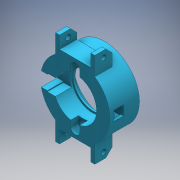
# Autodesk Inventor part: Tracking Bracelet
Saved by Autodesk Inventor 2016 (Build 200138000, 138)
## iProperties
Created: 2016-04-05
Part Number: Tracking Bracelet
Material: ABS Plastic
Document SubType Name: Modeling
Designer: xdlea
Density: 1.06 g/cm^3
Appearance: Turquoise
Author: xdlea
Autodesk Inventor part; units mm, degrees
ref_plane "YZ Plane" through (0, 0, 0) normal (1, 0, 0) x (0, 1, 0)
sketch "Sketch1" plane through (0, 0, 0) normal (0, 1, 0) x (-1, 0, 0)
  arc A0 (21.65, 4.5) -> (21.65, -4.5) centre (0, 0) ccw
  arc A1 (11.401069, 5.125) -> (11.401069, -5.125) centre (0, 0) ccw
  arc A2 (12.624381, 5.125) -> (12.624381, -5.125) centre (0, 0) ccw
  circle A3 centre (0, 0) radius 11.25 construction
  line L0 (10.014833, 5.125) -> (17.75, 5.125) construction
  line L1 (17.75, 5.125) -> (17.75, -5.125) construction
  line L2 (17.75, -5.125) -> (10.014833, -5.125) construction
  line L3 (10.014833, -5.125) -> (10.014833, 5.125) construction
  line L4 (17.75, 4.5) -> (21.65, 4.5) construction
  line L5 (21.65, 4.5) -> (21.65, -4.5) construction
  line L6 (21.65, -4.5) -> (17.75, -4.5) construction
  line L7 (17.75, -4.5) -> (17.75, 4.5) construction
  line L8 (-30.957812, 0) -> (30.957812, 0) construction
  arc A4 (19.602847, 4.5) -> (19.602847, -4.5) centre (0, 0) ccw
  line L9 (12.624381, 5.125) -> (17.75, 5.125)
  line L10 (17.75, 5.125) -> (17.75, 4.5)
  line L11 (17.75, 4.5) -> (19.602847, 4.5)
  line L12 (19.602847, 4.5) -> (21.65, 4.5)
  line L13 (21.65, -4.5) -> (19.602847, -4.5)
  line L14 (19.602847, -4.5) -> (17.75, -4.5)
  line L15 (17.75, -4.5) -> (17.75, -5.125)
  line L16 (17.75, -5.125) -> (12.624381, -5.125)
  line L17 (12.624381, 5.125) -> (11.401069, 5.125)
  line L18 (12.624381, -5.125) -> (11.401069, -5.125)
  arc A5 (11.401069, -5.125) -> (11.401069, 5.125) centre (0, 0) ccw
  arc A6 (12.624381, -5.125) -> (12.624381, 5.125) centre (0, 0) ccw
  arc A7 (19.602847, -4.5) -> (19.602847, 4.5) centre (0, 0) ccw
  arc A8 (21.65, -4.5) -> (21.65, 4.5) centre (0, 0) ccw
  line L19 (-21.908275, -3) -> (-19.908275, -3)
  line L20 (-19.908275, -3) -> (-19.908275, 3)
  line L21 (-19.908275, 3) -> (-21.908275, 3)
  line L22 (-21.908275, 3) -> (-21.908275, -3)
  line L23 (-19.908275, -4.6077) -> (-14.836045, -4.6077)
  line L24 (-14.836045, -4.6077) -> (-14.836045, 2.3923)
  line L25 (-14.836045, 2.3923) -> (-19.908275, 2.3923)
  line L26 (-19.908275, 2.3923) -> (-19.908275, -4.6077)
  dimension "d1" = 25
  dimension "d4" = 27.25
  dimension "d7" = 22.5
  dimension "d8" = 29
  dimension "d9" = 10.25
  dimension "d10" = 3.9
  dimension "d11" = 9
  dimension "d12" = 2
  dimension "d51" = 6
  dimension "d52" = 2
  dimension "d53" = 7
  constraints: 52 end point, 20 point on circle, 9 centre point, 8 parallel, 7 point on line, 6 coincident, 6 perpendicular, 4 horizontal, 3 collinear, 3 concentric, 1 other
  measures "d1" diameter of A1
  measures "d4" diameter of A2
  measures "d7" diameter of A3
  measures "d9" distance of L0.end L1.end
  measures "d10" distance of L5.end L6.end
  measures "d11" distance of L5.end L4.end
  measures "d12" radial gap between concentric circles of A0 A4
  measures "d51" distance between parallel lines of L21 L19
  measures "d52" distance of L19.start L19.end
  measures "d53" distance between parallel lines of L25 L23
sketch "Sketch1 outline for Extrusion3" plane through (0, 0, 0) normal (0, 1, 0) x (-1, 0, 0)
  circle A0 centre (0, 0) radius 22.112723
  circle A1 centre (0, 0) radius 20.112723
extrude "Extrusion3" add sketch "Sketch1 outline for Extrusion3" along normal blind 7.6
sketch "Sketch1 outline for Extrusion4" plane through (0, 0, 0) normal (0, 1, 0) x (-1, 0, 0)
  circle A0 centre (0, 0) radius 12.5
  circle A1 centre (0, 0) radius 20.112723
extrude "Extrusion4" add sketch "Sketch1 outline for Extrusion4" along normal blind 1.25
sketch "Sketch1 outline for Extrusion5" plane through (0, 0, 0) normal (0, 1, 0) x (-1, 0, 0)
  arc A0 (21.65, 4.5) -> (21.65, -4.5) centre (0, 0) ccw
  line L0 (21.65, -4.5) -> (17.75, -4.5)
  line L1 (17.75, -4.5) -> (17.75, -5.125)
  line L2 (17.75, -5.125) -> (12.624381, -5.125)
  arc A1 (12.624381, -5.125) -> (12.624381, 5.125) centre (0, 0) cw
  line L3 (12.624381, 5.125) -> (17.75, 5.125)
  line L4 (17.75, 5.125) -> (17.75, 4.5)
  line L5 (17.75, 4.5) -> (21.65, 4.5)
extrude "Extrusion5" add sketch "Sketch1 outline for Extrusion5" against normal blind 11.25
sketch "Sketch1 outline for Extrusion6" plane through (0, 0, 0) normal (0, 1, 0) x (-1, 0, 0)
  arc A0 (21.65, -4.5) -> (21.65, 4.5) centre (0, 0) ccw
  line L0 (21.65, 4.5) -> (17.75, 4.5)
  line L1 (17.75, 4.5) -> (17.75, 5.125)
  line L2 (17.75, 5.125) -> (12.624381, 5.125)
  arc A1 (12.624381, 5.125) -> (12.624381, -5.125) centre (0, 0) cw
  line L3 (12.624381, -5.125) -> (17.75, -5.125)
  line L4 (17.75, -5.125) -> (17.75, -4.5)
  line L5 (17.75, -4.5) -> (21.65, -4.5)
extrude "Extrusion6" add sketch "Sketch1 outline for Extrusion6" against normal blind 1
sketch "Sketch2" plane through (0, 1.25, 0) normal (0, 1, 0) x (1, 0, 0)
  circle A0 centre (0, 17) radius 2.425
  line L0 (30.957812, 0) -> (-30.957812, 0) construction
  line L1 (0, 42.7) -> (0, -42.7) construction
  point P0 (0, 0)
  dimension "d21" = 4.85
  dimension "d22" = 17
  constraints: 1 centre point, 1 point on line
  measures "d21" diameter of A0
  measures "d22" distance from line of L0 A0.centre
sketch "Sketch2 outline for Extrusion7" plane through (0, 1.25, 0) normal (0, 1, 0) x (1, 0, 0)
  circle A0 centre (0, 17) radius 2.425
extrude "Extrusion7" cut sketch "Sketch2 outline for Extrusion7" against normal blind 7.5
sketch "Sketch3" plane through (0, -6.25, -17) normal (0, 1, 0) x (1, 0, 0)
  arc A0 (2.875, 0) -> (-2.875, 0) centre (0, 0) ccw
  circle A1 centre (0, -34) radius 2.425
  circle A2 centre (0, 0) radius 2.425
  line L0 (-2.875, 0) -> (-2.875, -3.681779)
  arc A3 (-12.624381, -22.125) -> (-12.624381, -11.875) centre (0, -17) ccw
  line L1 (2.875, 0) -> (2.875, -3.681779)
  arc A4 (2.875, -3.681779) -> (-2.875, -3.681779) centre (0, -17) ccw
  dimension "d25" = 5.75
  constraints: 6 point on circle, 4 end point, 2 centre point, 2 concentric, 2 tangent, 1 parallel, 1 vertical
  measures "d25" diameter of A0
sketch "Sketch3 outline for Extrusion8" plane through (0, -6.25, -17) normal (0, 1, 0) x (1, 0, 0)
  arc A0 (2.875, 0) -> (-2.875, 0) centre (0, 0) ccw
  line L0 (2.875, -3.681779) -> (2.875, 0)
  arc A1 (-2.875, -3.681779) -> (2.875, -3.681779) centre (0, -17) cw
  line L1 (-2.875, 0) -> (-2.875, -3.681779)
extrude "Extrusion8" cut sketch "Sketch3 outline for Extrusion8" against normal blind 7.5
chamfer "Chamfer1" distance 3 angle 25 1 edges at (-2.425, 1.25, -17)
sketch "Sketch5" plane through (0, 0, 0) normal (1, 0, 0) x (0, 1, 0)
  line L0 (0, 42.7) -> (0, -42.7) construction
  line L1 (-48.962855, 0) -> (11.753777, 0) construction
  ellipse E0 centre (-14.482928, 0) end of major axis (3.017072, 0) minor radius 22.5 (-11.25, 22.112723) -> (-11.25, -22.112723) ccw
  line L2 (-11.25, 22.112723) -> (-11.25, -22.112723) construction
  ellipse E1 centre (-14.482928, 0) end of major axis (-14.482928, 30.5) minor radius 25.5 (3.079973, 22.112723) -> (3.079973, -22.112723) ccw
  line L3 (3.079973, -22.112723) -> (-11.25, -22.112723)
  line L4 (-11.25, 22.112723) -> (3.079973, 22.112723)
  spline S0 degree 5 poles (-9.370672, 29.888789) (-9.607667, 29.946061) (-9.845455, 30.000062) (-10.08398, 30.050769) (-13.432172, 30.714105) (-16.900715, 30.723992) (-20.090193, 30.119162) (-26.095525, 27.802909) (-31.037596, 23.674589) (-33.16656, 21.251032) (-36.759867, 15.847694) (-38.905719, 9.719856) (-39.623591, 6.515342) (-40.342276, 0) (-39.623591, -6.515342) (-38.905719, -9.719856) (-36.759867, -15.847694) (-33.16656, -21.251032) (-31.037596, -23.674589) (-26.095525, -27.802909) (-20.090193, -30.119162) (-16.900715, -30.723992) (-13.432172, -30.714105) (-10.08398, -30.050769) (-9.845455, -30.000062) (-9.607667, -29.946061) (-9.370672, -29.888789) knots 0 0 0 0 0 0 0.01237227 0.01237227 0.01237227 0.17318041 0.17318041 0.17318041 0.33468989 0.33468989 0.33468989 0.5 0.5 0.5 0.66531011 0.66531011 0.66531011 0.82681959 0.82681959 0.82681959 0.98762773 0.98762773 0.98762773 1 1 1 1 1 1 construction
  point P0 (0, 0)
  point P1 (-11.25, -4.5)
  point P2 (-11.25, 4.5)
  dimension "d39" = 8
  dimension "d40" = 22.5
  dimension "d41" = 17.5
  dimension "d42" = 30.5
  dimension "d43" = 25.5
  constraints: 4 end point, 3 point on line, 1 coincident, 1 parallel, 1 perpendicular, 1 vertical alignment, 13 other
pattern_circular "Circular Pattern2" count 2 over 360 about axis through (0, 0, 0) along (0, -1, 0) of "Extrusion7", "Extrusion8", "Chamfer1"
ref_plane "Work Plane1" through (22.112723, 0, 0) normal (1, 0, 0) x (0, 1, 0)
sketch "Sketch8" plane through (22.112723, 0, 0) normal (1, 0, 0) x (0, 1, 0)
  line L0 (-8.575, 3.075) -> (-2.425, 3.075)
  line L1 (-2.425, 3.075) -> (-2.425, -3.075)
  line L2 (-2.425, -3.075) -> (-8.575, -3.075)
  line L3 (-8.575, -3.075) -> (-8.575, 3.075)
  line L4 (-8.575, 3.075) -> (-2.425, -3.075) construction
  line L5 (-2.425, 3.075) -> (-8.575, -3.075) construction
  line L6 (-15.02, 0) -> (11.37, 0) construction
  line L7 (0, 30.957812) -> (0, -30.957812) construction
  point P0 (0, 0)
  point P1 (-5.5, 0)
  dimension "d54" = 6.15
  dimension "d55" = 6.15
  dimension "d56" = 5.5
  constraints: 12 end point, 2 midpoint, 2 parallel, 1 horizontal, 1 perpendicular, 1 point on line
  measures "d54" distance of L0.end L1.end
  measures "d55" distance of L1.end L2.end
  measures "d56" distance from line of point (-5.5, 0) L7
sketch "Sketch8 outline for Extrusion11" plane through (22.112723, 0, 0) normal (1, 0, 0) x (0, 1, 0)
  line L0 (-8.575, 3.075) -> (-2.425, 3.075)
  line L1 (-2.425, 3.075) -> (-2.425, -3.075)
  line L2 (-2.425, -3.075) -> (-8.575, -3.075)
  line L3 (-8.575, -3.075) -> (-8.575, 3.075)
extrude "Extrusion11" cut sketch "Sketch8 outline for Extrusion11" against normal up to next
ref_plane "Work Plane2" through (20.112723, 0, 0) normal (1, 0, 0) x (0, 1, 0)
sketch "Sketch9" plane through (20.112723, 0, 0) normal (1, 0, 0) x (0, 1, 0)
  line L0 (-8.575, 3.75) -> (-2.425, 3.75)
  line L1 (-2.425, 3.75) -> (-2.425, -3.75)
  line L2 (-2.425, -3.75) -> (-8.575, -3.75)
  line L3 (-8.575, -3.75) -> (-8.575, 3.75)
  line L4 (-8.575, 3.75) -> (-2.425, -3.75) construction
  line L5 (-2.425, 3.75) -> (-8.575, -3.75) construction
  line L6 (-2.425, 3.075) -> (-2.425, -3.075) construction
  line L7 (-8.575, -3.075) -> (-2.425, -3.075) construction
  line L8 (-2.425, 3.075) -> (-8.575, 3.075) construction
  line L9 (-8.575, -3.075) -> (-8.575, 3.075) construction
  point P0 (0, 0)
  point P1 (-5.5, 0)
  point P2 (-5.5, 0)
  dimension "d60" = 7.5
  constraints: 12 end point, 3 midpoint, 2 collinear, 2 parallel, 1 horizontal, 1 horizontal alignment, 1 perpendicular
  measures "d60" distance of L0.end L1.end
sketch "Sketch9 outline for Extrusion12" plane through (20.112723, 0, 0) normal (1, 0, 0) x (0, 1, 0)
  line L0 (-8.575, 3.75) -> (-2.425, 3.75)
  line L1 (-2.425, 3.75) -> (-2.425, -3.75)
  line L2 (-2.425, -3.75) -> (-8.575, -3.75)
  line L3 (-8.575, -3.75) -> (-8.575, 3.75)
extrude "Extrusion12" cut sketch "Sketch9 outline for Extrusion12" against normal up to next
sketch "Sketch10" plane through (0, 0, 0) normal (1, 0, 0) x (0, 1, 0)
  line L0 (-11.25, 22.112723) -> (-11.25, -22.112723) construction
  line L1 (-11.25, -22.112723) -> (-0.25, -22.112723)
  line L2 (-0.25, -22.112723) -> (-0.25, -30.112723)
  line L3 (-0.25, -30.112723) -> (-11.25, -30.112723)
  line L4 (-11.25, -30.112723) -> (-11.25, -22.112723)
  circle A0 centre (-5.75, -26.112723) radius 1.575
  point P0 (0, 0)
  point P1 (-11.25, -4.5)
  point P2 (-11.25, 4.5)
  dimension "d63" = 8
  dimension "d64" = 11
  dimension "d65" = 3.15
  constraints: 8 end point, 2 parallel, 1 centre point, 1 horizontal, 1 perpendicular
  measures "d63" distance of L1.end L2.end
  measures "d64" distance of L2.end L3.end
  measures "d65" diameter of A0
sketch "Sketch10 outline for Extrusion13" plane through (0, 0, 0) normal (1, 0, 0) x (0, 1, 0)
  line L0 (-11.25, -22.112723) -> (-0.25, -22.112723)
  line L1 (-11.25, -30.112723) -> (-11.25, -22.112723)
  line L2 (-0.25, -22.112723) -> (-0.25, -30.112723)
  line L3 (-0.25, -30.112723) -> (-11.25, -30.112723)
  circle A0 centre (-5.75, -26.112723) radius 1.575
extrude "Extrusion13" add sketch "Sketch10 outline for Extrusion13" along normal mid plane 25
sketch "Sketch11" plane through (-12.5, -0.25, -22.112723) normal (0, 0, 1) x (1, 0, 0)
  line L0 (12.5, -11) -> (12.5, 0) projected
  line L1 (12.5, 0) -> (0, 0) projected
  line L2 (0, -11) -> (0, 0) projected
  line L3 (0, -11) -> (12.5, -11) projected
  line L4 (12.5, -11) -> (25, -11) projected
  line L5 (25, 0) -> (25, -11) projected
  line L6 (25, 0) -> (12.5, 0) projected
  point P0 (12.5, 0.25)
sketch "Sketch11 outline for Extrusion14" plane through (-12.5, -0.25, -22.112723) normal (0, 0, 1) x (1, 0, 0)
  line L0 (25, 0) -> (0, 0)
  line L1 (0, 0) -> (0, -11)
  line L2 (0, -11) -> (25, -11)
  line L3 (25, -11) -> (25, 0)
extrude "Extrusion14" add sketch "Sketch11 outline for Extrusion14" along normal up to next
sketch "Sketch10 outline for Extrusion15" plane through (0, 0, 0) normal (1, 0, 0) x (0, 1, 0)
  line L0 (-11.25, -22.112723) -> (-0.25, -22.112723)
  line L1 (-11.25, -30.112723) -> (-11.25, -22.112723)
  line L2 (-0.25, -22.112723) -> (-0.25, -30.112723)
  line L3 (-0.25, -30.112723) -> (-11.25, -30.112723)
  circle A0 centre (-5.75, -26.112723) radius 1.575
extrude "Extrusion15" cut sketch "Sketch10 outline for Extrusion15" along normal mid plane 20
chamfer "Chamfer2" distance 4 angle 45 2 edges at (11.25, -0.25, -30.1127) (-11.25, -0.25, -30.1127)
pattern_circular "Circular Pattern3" count 2 over 360 about axis through (0, 0, 0) along (0, -1, 0) of "Extrusion13", "Extrusion14", "Extrusion15", "Chamfer2"
equation "\"d42\" = d40 + d39"
equation "\"d43\" = d41 + d39"
equation "\"d55\" = d54"
body "Solid2"
